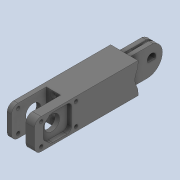
# Autodesk Inventor part: L1Index
Saved by Autodesk Inventor 2020 (Build 240168000, 168)
## iProperties
Created: 2020-01-19
Part Number: L1Index
Material: Generic
Document SubType Name: Modeling
Designer: sami_
Density: 1 g/cm^3
Appearance: Gray
Author: sami_
Autodesk Inventor part; units mm, degrees
ref_plane "YZ Plane" through (0, 0, 0) normal (1, 0, 0) x (0, 1, 0)
ref_plane "XZ Plane" through (0, 0, 0) normal (0, 1, 0) x (-1, 0, 0)
ref_plane "XY Plane" through (0, 0, 0) normal (0, 0, 1) x (1, 0, 0)
sketch "Sketch1" plane through (0, 0, 0) normal (0, 1, 0) x (-1, 0, 0)
  line L0 (-3.0814, 0) -> (-5.0814, 0)
  line L1 (-8.0814, 0) -> (-8.0814, -16)
  line L2 (-8.0814, -16) -> (-6.0814, -16)
  line L3 (-3.0814, -16) -> (-3.0814, 0)
  line L4 (-3.0814, 0) -> (-5.0814, 0)
  line L5 (-5.0814, 0) -> (-5.0814, -16)
  line L6 (-5.0814, -16) -> (-3.0814, -16)
  line L7 (-3.0814, -16) -> (-3.0814, 0)
  line L8 (-8.0814, -16) -> (-6.0814, -16)
  line L9 (-6.0814, -16) -> (-6.0814, 0)
  line L10 (-6.0814, 0) -> (-8.0814, 0)
  line L11 (-8.0814, 0) -> (-8.0814, -16)
  line L12 (-5.0814, 0) -> (-6.0814, 0) construction
  line L13 (-6.0814, 0) -> (-8.0814, 0)
  line L14 (-5.0814, -16) -> (-3.0814, -16)
  line L15 (-6.0814, -16) -> (-5.0814, -16) construction
  line L16 (-12.8814, 0) -> (-0.2814, 0)
  line L17 (-0.2814, 0) -> (-0.2814, 31.613)
  line L18 (-0.2814, 31.613) -> (-12.8814, 31.613)
  line L19 (-12.8814, 31.613) -> (-12.8814, 0)
  line L20 (-5.5814, -16) -> (-5.5814, 34) construction
  line L21 (-0.2814, 47.613) -> (-2.2814, 47.613)
  line L22 (-2.2814, 47.613) -> (-2.2814, 31.613)
  line L23 (-2.2814, 31.613) -> (-0.2814, 31.613)
  line L24 (-0.2814, 31.613) -> (-0.2814, 47.613)
  line L25 (-12.8814, 31.613) -> (-8.8814, 31.613)
  line L26 (-8.8814, 31.613) -> (-8.8814, 47.613)
  line L27 (-8.8814, 47.613) -> (-12.8814, 47.613)
  line L28 (-12.8814, 47.613) -> (-12.8814, 31.613)
  line L29 (-12.8814, 37.613) -> (-0.2814, 37.613) construction
  line L30 (-8.0814, -11) -> (-3.0814, -11) construction
  line L31 (-3.0814, -5) -> (-8.0814, -5)
  point P0 (-6.0814, -5)
  point P1 (-5.0814, -5)
  dimension "d11" = 16
  dimension "d12" = 5
  dimension "d13" = 2
  dimension "d14" = 16
  dimension "d15" = 2
  dimension "d16" = 16
  dimension "d17" = 50
  dimension "d18" = 2
  dimension "d19" = 4
  dimension "d20" = 6.6
  dimension "d21" = 3.3
  dimension "d22" = 16
  dimension "d24" = 6
  dimension "d26" = 5
  dimension "d28" = 6
  dimension "d29" = 36.613
  dimension "d155" = 48.613
  constraints: 64 end point, 11 parallel, 11 perpendicular, 6 collinear, 6 point on line, 3 horizontal, 1 midpoint, 1 vertical
  measures "d11" distance of L1.end L1.start
  measures "d12" distance of L1.end L3.start
  measures "d13" distance of L6.end L5.end
  measures "d14" distance of L5.end L0.end
  measures "d15" distance of L10.end L9.end
  measures "d16" distance of L9.end L2.end
  measures "d17" distance of L20.start L20.end
  measures "d18" distance between parallel lines of L24 L22
  measures "d19" distance between parallel lines of L28 L26
  measures "d20" distance between parallel lines of L26 L22
  measures "d21" distance between parallel lines of L20 L26
  measures "d22" distance of L25.end L26.end
  measures "d24" distance between parallel lines of L25 L29
  measures "d26" distance between parallel lines of L6 L30
  measures "d28" distance between parallel lines of L31 L30
  measures "d29" distance between parallel lines of L18 L31
  measures "d155" distance between parallel lines of L30 L29
extrude "Extrusion1" add sketch "Sketch1" along normal blind 14
sketch "Sketch7" plane through (5.0814, 0, -5) normal (1, 0, 0) x (0, 0, -1)
  circle A0 centre (6, 7) radius 5
  line L0 (-5, 0) -> (11, 0) projected
  line L1 (-5, 14) -> (11, 14) projected
  line L2 (11, 0) -> (11, 14) projected
  line L3 (0, 0) -> (0, 14) projected
  dimension "d65" = 10
  dimension "d67" = 7
  dimension "d69" = 6
  constraints: 1 centre point
  measures "d65" diameter of A0
  measures "d67" distance from line of L1 A0.centre
  measures "d69" distance from line of L3 A0.centre
extrude "Extrusion5" add sketch "Sketch7" along normal up to surface (1 mm away) contours A0
sketch "Sketch2" plane through (2.2814, 0, 47.613) normal (1, 0, 0) x (0, 0, -1)
  circle A0 centre (10, 7) radius 3.5
  line L0 (16, 0) -> (16, 14) projected
  line L1 (0, 0) -> (16, 0) projected
  point P0 (47.613, 0)
  dimension "d32" = 7
  dimension "d33" = 6
  dimension "d34" = 7
  constraints: 1 centre point
  measures "d32" diameter of A0
  measures "d33" distance from line of L0 A0.centre
  measures "d34" distance from line of L1 A0.centre
extrude "Extrusion2" cut sketch "Sketch2" along normal through all both and the other way through all
sketch "Sketch3" plane through (8.0814, 0, 0) normal (1, 0, 0) x (0, 0, -1)
  circle A0 centre (11, 7) radius 2
  line L0 (0, 0) -> (16, 0) projected
  line L1 (16, 0) -> (16, 14) projected
  line L2 (12.7321, 6) -> (9.2679, 6)
  dimension "d37" = 4
  dimension "d38" = 7
  dimension "d39" = 5
  dimension "d42" = 1
  constraints: 2 end point, 2 point on circle, 1 centre point, 1 horizontal
  measures "d37" diameter of A0
  measures "d38" distance from line of L0 A0.centre
  measures "d39" distance from line of L1 A0.centre
  measures "d42" distance centre to line of A0 L2
extrude "Extrusion3" cut sketch "Sketch3" against normal mid plane 14 contours A0 L2 picked at (11.0553, 7.2513)
sketch "Sketch4" plane through (12.8814, 0, 47.613) normal (1, 0, 0) x (0, 0, -1)
  line L0 (16.4999, 2.5) -> (16.4999, 3.7175) construction
  line L1 (16.4999, 3.7175) -> (16.9479, 4.0312) construction
  line L2 (16.9479, 4.0312) -> (18.2298, 4.0312) construction
  line L3 (18.2298, 4.0312) -> (18.2298, 4.9288) construction
  line L4 (18.2298, 4.9288) -> (17.035, 4.9288) construction
  line L5 (17.035, 4.9288) -> (16.4999, 5.1919) construction
  line L6 (16.4999, 5.1919) -> (16.4999, 6.3096) construction
  line L7 (16.4999, 6.3096) -> (17.035, 6.5728) construction
  line L8 (17.035, 6.5728) -> (18.2298, 6.5728) construction
  line L9 (18.2298, 6.5728) -> (18.2298, 7.4703) construction
  line L10 (18.2298, 7.4703) -> (16.9479, 7.4703) construction
  line L11 (16.9479, 7.4703) -> (16.4999, 7.784) construction
  line L12 (16.4999, 7.784) -> (16.4999, 8.8082) construction
  line L13 (16.4999, 8.8082) -> (17.035, 9.0713) construction
  line L14 (17.035, 9.0713) -> (18.2298, 9.0713) construction
  line L15 (18.2298, 9.0713) -> (18.2298, 9.9689) construction
  line L16 (18.2298, 9.9689) -> (16.9479, 9.9689) construction
  line L17 (16.9479, 9.9689) -> (16.4999, 10.2826) construction
  line L18 (16.4999, 10.2826) -> (16.4999, 11.5) construction
  line L19 (16.4999, 11.5) -> (15.4999, 12.5) construction
  line L20 (15.4999, 12.5) -> (8.0752, 12.5) construction
  line L21 (8.0752, 12.5) -> (4.4999, 9.5) construction
  line L22 (4.4999, 9.5) -> (4.4999, 7.4703) construction
  line L23 (4.4999, 7.4703) -> (3.3809, 7.4703) construction
  line L24 (3.3809, 7.4703) -> (3.3809, 6.5728) construction
  line L25 (3.3809, 6.5728) -> (4.4999, 6.5728) construction
  line L26 (4.4999, 6.5728) -> (4.4999, 4.5) construction
  line L27 (4.4999, 4.5) -> (8.0752, 1.5) construction
  line L28 (8.0752, 1.5) -> (15.4999, 1.5) construction
  line L29 (15.4999, 1.5) -> (16.4999, 2.5) construction
  circle A0 centre (9.9999, 7) radius 2 construction
  circle A1 centre (10, 7) radius 3.5 construction
  circle A2 centre (10, 7) radius 3.5 construction
  line L30 (17, 13) -> (4, 13)
  line L31 (4, 13) -> (4, 1)
  line L32 (4, 1) -> (17, 1)
  line L33 (17, 1) -> (17, 13)
  line L34 (7.5, 13) -> (4, 10)
  line L35 (47.613, 0) -> (47.613, 14) projected
  line L36 (47.613, 7) -> (0, 7) construction
  line L37 (0, 0) -> (0, 14) projected
  line L38 (0, 0) -> (47.613, 0) projected
  line L39 (7.5, 1) -> (4, 4)
  line L40 (47.613, 14) -> (0, 14)
  line L41 (0, 14) -> (0, 0)
  line L42 (0, 0) -> (47.613, 0)
  line L43 (47.613, 0) -> (47.613, 14)
  dimension "d43" = 6.619
  dimension "d44" = 6.5
  dimension "d45" = 11
  dimension "d46" = 12
  dimension "d47" = 12
  dimension "d48" = 13
  dimension "d49" = 5.5001
  dimension "d50" = 6.4999
  dimension "d51" = 7
  dimension "d54" = 6
  dimension "d56" = 3
  dimension "d57" = 3.5
  dimension "d58" = 7
  dimension "d59" = 3
  dimension "d60" = 3.5
  constraints: 82 end point, 4 parallel, 4 point on line, 2 centre point, 2 horizontal, 2 midpoint, 2 perpendicular, 1 coincident
  measures "d43" distance from line of L24 A0.centre
  measures "d44" distance from line of L12 A0.centre
  measures "d45" distance between parallel lines of L28 L20
  measures "d46" distance of L31.end L30.end
  measures "d47" distance between parallel lines of L26 L6
  measures "d48" distance between parallel lines of L33 L31
  measures "d49" distance from line of L26 A2.centre
  measures "d50" distance from line of L6 A2.centre
  measures "d51" distance from line of A2.centre L33
  measures "d54" distance from line of L30 A2.centre
  measures "d56" distance of L30.end L34.end
  measures "d57" distance of L30.end L34.start
  measures "d58" distance between parallel lines of L38 L36
  measures "d59" distance of L31.end L39.end
  measures "d60" distance of L31.end L39.start
extrude "Extrusion4" cut sketch "Sketch4" against normal blind 2 contours L33 L32 L39 L31 L34 L30
fillet "Fillet1" radius 2 4 edges at (11.8814, 4, 43.613) (11.8814, 10, 43.613) (11.8814, 1, 30.613) (11.8814, 13, 30.613)
fillet "Fillet2" radius 2 2 edges at (11.8814, 1, 40.113) (11.8814, 13, 40.113)
sketch "Sketch8" plane through (12.8814, 0, 47.613) normal (1, 0, 0) x (0, 0, -1)
  circle A0 centre (19, 12) radius 0.8
  circle A1 centre (19, 2) radius 0.8
  circle A2 centre (3, 12) radius 0.8
  circle A3 centre (3, 2) radius 0.8
  line L0 (0, 0) -> (0, 14) projected
  line L1 (0, 0) -> (47.613, 0) projected
  line L2 (0, 14) -> (47.613, 14) projected
  dimension "d72" = 1.6
  dimension "d73" = 1.6
  dimension "d74" = 1.6
  dimension "d75" = 1.6
  dimension "d77" = 16
  dimension "d78" = 16
  dimension "d79" = 3
  dimension "d80" = 2
  dimension "d81" = 2
  dimension "d82" = 2
  dimension "d83" = 2
  dimension "d84" = 3
  constraints: 4 centre point
  measures "d72" diameter of A0
  measures "d73" diameter of A1
  measures "d74" diameter of A2
  measures "d75" diameter of A3
  measures "d77" distance of A2.centre A0.centre
  measures "d78" distance of A3.centre A1.centre
  measures "d79" distance from line of L0 A3.centre
  measures "d80" distance from line of L1 A3.centre
  measures "d81" distance from line of L1 A1.centre
  measures "d82" distance from line of L2 A0.centre
  measures "d83" distance from line of L2 A2.centre
  measures "d84" distance from line of L0 A2.centre
extrude "Extrusion6" cut sketch "Sketch8" against normal blind 4
sketch "Sketch15" plane through (0.2814, 0, 0) normal (-1, 0, 0) x (0, 0, 1)
  circle A0 centre (28.613, 12) radius 0.8
  circle A1 centre (28.613, 2) radius 0.8
  circle A2 centre (44.613, 2) radius 0.8
  circle A3 centre (44.613, 12) radius 0.8
  line L0 (0, 14) -> (47.613, 14) projected
  line L1 (47.613, 0) -> (47.613, 14) projected
  line L2 (0, 0) -> (47.613, 0) projected
  dimension "d129" = 1.6
  dimension "d130" = 1.6
  dimension "d131" = 1.6
  dimension "d132" = 1.6
  dimension "d133" = 16
  dimension "d134" = 2
  dimension "d135" = 2
  dimension "d136" = 3
  dimension "d137" = 2
  dimension "d138" = 16
  dimension "d139" = 3
  dimension "d140" = 2
  constraints: 4 centre point
  measures "d129" diameter of A0
  measures "d130" diameter of A1
  measures "d131" diameter of A2
  measures "d132" diameter of A3
  measures "d133" distance of A3.centre A0.centre
  measures "d134" distance from line of L0 A0.centre
  measures "d135" distance from line of L0 A3.centre
  measures "d136" distance from line of L1 A3.centre
  measures "d137" distance from line of L2 A1.centre
  measures "d138" distance of A2.centre A1.centre
  measures "d139" distance from line of L1 A2.centre
  measures "d140" distance from line of L2 A2.centre
extrude "Extrusion11" cut sketch "Sketch15" against normal blind 4
fillet "Fillet3" radius 3 4 edges at (10.8814, 14, 47.613) (10.8814, 0, 47.613) (1.2814, 14, 47.613) (1.2814, 0, 47.613)
fillet "Fillet4" radius 7 4 edges at (7.0814, 0, -16) (7.0814, 14, -16) (4.0814, 14, -16) (4.0814, 0, -16)
sketch "Sketch9" plane through (12.8814, 0, 0) normal (1, 0, 0) x (0, 0, -1)
  line L0 (0, 0) -> (0, 14) projected
  line L1 (0, 7) -> (-1.5, 7)
  arc A0 (-1.5, 7) -> (0, 3.2919) centre (3.8333, 7) ccw
  arc A1 (0, 10.7081) -> (-1.5, 7) centre (3.8333, 7) ccw
  dimension "d89" = 1.5
  dimension "d90" = 4
  dimension "d91" = 4
  constraints: 4 point on circle, 2 centre point, 2 end point, 2 point on line, 1 coincident, 1 concentric, 1 horizontal, 1 midpoint
  measures "d89" distance of L1.start L1.end
  measures "d90" distance of L1.end A0.end
  measures "d91" distance of L1.end A1.start
extrude "Extrusion7" cut sketch "Sketch9" against normal up to surface (4.8 mm away)
fillet "Fillet5" radius 7 2 edges at (10.4814, 3.2919, 0) (10.4814, 10.7081, 0)
sketch "Sketch10" plane through (0.2814, 0, 0) normal (-1, 0, 0) x (0, 0, 1)
  line L0 (0, 0) -> (0, 14)
  line L1 (0, 7) -> (-1.5, 7) construction
  arc A0 (-1.5, 7) -> (0, 3.2919) centre (3.8333, 7) ccw construction
  arc A1 (0, 10.7081) -> (-1.5, 7) centre (3.8333, 7) ccw construction
  line L2 (0, 7) -> (1.5, 7)
  arc A2 (0, 3.2919) -> (1.5, 7) centre (-3.8333, 7) ccw
  arc A3 (1.5, 7) -> (0, 10.7081) centre (-3.8333, 7) ccw
  point P0 (0, 0)
  dimension "d95" = 1.5
  dimension "d96" = 4
  dimension "d97" = 4
  constraints: 8 point on circle, 6 end point, 4 centre point, 3 symmetric about line, 2 coincident, 2 point on line, 1 concentric, 1 horizontal, 1 midpoint, 2 other
  measures "d95" distance of L1.start L1.end
  measures "d96" distance of L1.end A0.end
  measures "d97" distance of L1.end A1.start
extrude "Extrusion8" cut sketch "Sketch10" against normal up to surface (2.8 mm away)
fillet "Fillet6" radius 7 2 edges at (1.6814, 3.2919, 0) (1.6814, 10.7081, 0)
sketch "Sketch11" plane through (2.2814, 0, 31.613) normal (0, 0, 1) x (1, 0, 0)
  line L0 (0, 0) -> (6.6, 0) construction
  line L1 (6.6, 0) -> (6.6, 14) construction
  line L2 (0, 0) -> (6.6, 0) construction
  line L3 (6.6, 0) -> (6.6, 14) construction
  line L4 (6.6, 14) -> (0, 14) construction
  line L5 (0, 14) -> (0, 0) construction
  line L6 (0, 14) -> (6.6, 14) construction
  line L7 (3.3, 14) -> (3.3, 0) construction
  line L8 (3.3, 7) -> (0, 7) construction
  line L9 (0, 0) -> (0, 14) projected
  circle A0 centre (3.3, 5.25) radius 0.6
  circle A1 centre (3.3, 8.75) radius 0.6
  point P0 (-2.2814, 0)
  dimension "d101" = 6.6
  dimension "d102" = 3.3
  dimension "d103" = 14
  dimension "d104" = 7
  dimension "d105" = 1.2
  dimension "d106" = 1.2
  dimension "d107" = 1.75
  dimension "d108" = 1.75
  constraints: 12 end point, 4 midpoint, 2 centre point, 2 parallel, 2 point on line, 1 horizontal, 1 perpendicular
  measures "d101" distance between parallel lines of L5 L1
  measures "d102" distance between parallel lines of L5 L7
  measures "d103" distance of L0.start L4.end
  measures "d104" distance between parallel lines of L0 L8
  measures "d105" diameter of A0
  measures "d106" diameter of A1
  measures "d107" distance from line of L8 A1.centre
  measures "d108" distance from line of L8 A0.centre
extrude "Extrusion9" cut sketch "Sketch11" against normal up to surface (36.613 mm away)
fillet "Fillet7" radius 1 4 edges at (5.5814, 4.65, -5) (5.5814, 9.35, -5) (4.9814, 5.25, 31.613) (4.9814, 8.75, 31.613)
sketch "Sketch16" plane through (8.0814, 0, 0) normal (1, 0, 0) x (0, 0, -1)
  arc A0 (9, 0) -> (9, 14) centre (9, 7) ccw projected
  arc A1 (16, 7) -> (11.6755, 12.5045) centre (10.2792, 6.9565) ccw
  line L0 (11.6755, 12.5045) -> (-0.0109, 12.5045)
  arc A2 (-0.8514, 9.5492) -> (0, 12.8949) centre (-7, 12.8949) ccw projected
  line L1 (11.6755, 12.5045) -> (23.362, 12.5045) construction
  line L2 (-0.0109, 12.5045) -> (-0.0109, 16.8803)
  line L3 (-0.0109, 16.8803) -> (16, 16.8803)
  line L4 (16, 16.8803) -> (16, 7)
  point P0 (0, 0)
  dimension "d143" = 7
  dimension "d144" = 180
  constraints: 10 end point, 4 point on circle, 3 perpendicular, 1 centre point, 1 collinear, 1 horizontal, 1 tangent
  measures "d143" distance of L4.end L0.start
  measures "d144" angle of L0 L1
extrude "Extrusion12" cut sketch "Sketch16" against normal blind 10
sketch "Sketch17" plane through (2.2814, 0, 31.613) normal (0, 0, 1) x (1, 0, 0)
  circle A0 centre (3.3, 1.75) radius 0.6
  circle A1 centre (3.3, 12.25) radius 0.6
  circle A2 centre (3.3, 8.75) radius 0.6 projected
  circle A3 centre (3.3, 5.25) radius 0.6 projected
  point P0 (-2.2814, 0)
  dimension "d147" = 1.2
  dimension "d149" = 3.5
  dimension "d150" = 3.5
  dimension "d151" = 1.2
  constraints: 2 centre point
  measures "d147" diameter of A1
  measures "d149" distance of A2.centre A1.centre
  measures "d150" distance of A3.centre A0.centre
  measures "d151" diameter of A0
extrude "Extrusion13" cut sketch "Sketch17" against normal up to surface (36.613 mm away) contours A0 | A1
fillet "Fillet8" radius 1 2 edges at (4.9814, 1.75, 31.613) (4.9814, 12.25, 31.613)
equation "\"d11\" = insideLength"
equation "\"d12\" = insideWidth"
equation "\"d13\" = insideThickness"
equation "\"d14\" = insideLength"
equation "\"d15\" = insideThickness"
equation "\"d16\" = insideLength"
equation "\"d18\" = LwingThickness"
equation "\"d19\" = RwingThickness"
equation "\"d20\" = winginsidewidth"
equation "\"d21\" = 0.5 * winginsidewidth"
equation "\"d22\" = wingLength"
equation "\"d30\" = midDepth"
equation "\"d65\" = pulleyDiameter"
equation "\"d67\" = 0.5 * midDepth"
equation "\"d32\" = bearingOutDiameter"
equation "\"d34\" = 0.5 * midDepth"
equation "\"d37\" = ShaftDiameter"
equation "\"d38\" = 0.5 * midDepth"
equation "\"d40\" = midDepth"
equation "\"d54\" = 0.5 * d46"
equation "\"d59\" = d56"
equation "\"d60\" = d57"
equation "\"d61\" = sensordepth"
equation "\"d72\" = d75"
equation "\"d73\" = d75"
equation "\"d74\" = d75"
equation "\"d88\" = 0.5 * midDepth"
equation "\"d94\" = 0.5 * midDepth"
equation "\"d98\" = sensordepth"
equation "\"d100\" = 0.5 * midDepth"
equation "\"insideLength\" = 16"
equation "\"insideThickness\" = 2"
equation "\"cableWidth\" = 1"
equation "\"insideWidth\" = 2 * insideThickness + cableWidth"
equation "\"midLength\" = 18.98592"
equation "\"wingLength\" = insideLength"
equation "\"LwingThickness\" = bearingthickness"
equation "\"RwingThickness\" = bearingthickness + sensordepth"
equation "\"bearingthickness\" = 2"
equation "\"sensordepth\" = 2"
equation "\"winginsidewidth\" = insideWidth + 2 * washerThickness"
equation "\"washerThickness\" = 0.8"
equation "\"SectionLength\" = 30.98592"
equation "\"insideholedistance\" = 6"
equation "\"midDepth\" = 14"
equation "\"bearingOutDiameter\" = 7"
equation "\"ShaftDiameter\" = 4"
equation "\"pulleyDiameter\" = 10"
equation "\"cableholediameter\" = 1.2"
body "Solid1"
